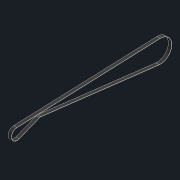
# Autodesk Inventor part: belt_2
Saved by Autodesk Inventor 2021 (Build 250183000, 183)
## iProperties
Created: 2021-07-18
Part Number: belt_2
Material: ゴム
Document SubType Name: Modeling
Designer: yuta0
Density: 0.93 g/cm^3
Appearance: ゴム - 黒
Mass: 7.90823 g
Surface Area: 229.594 cm^2
Volume: 8.50347 cm^3
購入先: ミスミ
在庫数: 0.0
Author: yuta0
Autodesk Inventor part; units mm, degrees
ref_plane "YZ Plane" through (0, 0, 0) normal (1, 0, 0) x (0, 1, 0)
ref_plane "XZ Plane" through (0, 0, 0) normal (0, 1, 0) x (-1, 0, 0)
ref_plane "XY Plane" through (0, 0, 0) normal (0, 0, 1) x (1, 0, 0)
sketch "スケッチ1" plane through (0, 0, 0) normal (1, 0, 0) x (0, 1, 0)
  arc A0 (17.1756, 0.6715) -> (-15.9786, -6.3353) centre (0, 0) ccw
  arc A1 (-34.1332, -435.9093) -> (34.3512, -438.657) centre (0, -440) ccw
  arc A2 (9.3592, -73.0018) -> (8.8263, -68.897) centre (1, -72) ccw
  line L0 (8.8263, -68.897) -> (-15.9786, -6.3353)
  line L1 (34.3512, -438.657) -> (17.1756, 0.6715)
  line L2 (9.3592, -73.0018) -> (-34.1332, -435.9093)
  arc A3 (17.5943, 0.6879) -> (-16.3681, -6.4898) centre (0, 0) ccw
  line L3 (-16.3681, -6.4898) -> (8.4368, -69.0514)
  arc A4 (8.9432, -72.9519) -> (8.4368, -69.0514) centre (1, -72) ccw
  line L4 (8.9432, -72.9519) -> (-34.5492, -435.8595)
  arc A5 (-34.5492, -435.8595) -> (34.7699, -438.6407) centre (0, -440) ccw
  line L5 (34.7699, -438.6407) -> (17.5943, 0.6879)
  arc A6 (16.7949, 0.6566) -> (-15.6244, -6.1949) centre (0, 0) ccw
  line L6 (-15.6244, -6.1949) -> (9.1805, -68.7565)
  arc A7 (9.7375, -73.0471) -> (9.1805, -68.7565) centre (1, -72) ccw
  line L7 (9.7375, -73.0471) -> (-33.7549, -435.9547)
  arc A8 (-33.7549, -435.9547) -> (33.9705, -438.6719) centre (0, -440) ccw
  line L8 (33.9705, -438.6719) -> (16.7949, 0.6566)
  dimension "d0" = 34.3775
  dimension "d1" = 68.7549
  dimension "d2" = 440
  dimension "d24" = 0.419
  dimension "d25" = 8
  dimension "d26" = 72
  dimension "d27" = 0.8
  dimension "d32" = 1
  constraints: 18 end point, 18 point on circle, 9 centre point, 6 tangent, 1 coincident, 1 vertical alignment, 10 other
  measures "d0" diameter of A0
  measures "d1" diameter of A1
  measures "d2" distance of A0.centre A1.centre
  measures "d24" distance between parallel lines of L1 L5
  measures "d25" radius of A4
  measures "d26" vertical distance of point (0, 0) A2.centre
  measures "d27" distance between parallel lines of L5 L8
  measures "d32" horizontal distance of point (0, 0) A2.centre
extrude "押し出し1" add sketch "スケッチ1" along normal mid plane 10 contours L1 A1 L2 A2 L0 A0 | L5 A5 L4 A4 L3 A3
